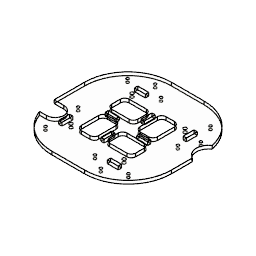
BasePlate_v8 (Autodesk Fusion 360 design; units mm, degrees)
Autodesk Fusion 360 part; units mm, degrees
sketch "Sketch1" plane through (0, 0, 0) normal (0, 0, 1) x (1, 0, 0)
  line L0 (-33.4, -17.4) -> (-33.4, 33.4) construction
  line L1 (-33.4, 33.4) -> (-27.4, 33.4) construction
  line L2 (-33.4, -17.4) -> (-36.4, -17.4)
  line L3 (-36.4, -17.4) -> (-36.4, -27.4)
  line L4 (-36.4, -27.4) -> (-33.4, -27.4)
  line L5 (-33.4, -27.4) -> (-33.4, -17.4)
  line L6 (-27.4, 33.4) -> (-17.4, 33.4)
  line L7 (-17.4, 33.4) -> (-17.4, 36.4)
  line L8 (-17.4, 36.4) -> (-27.4, 36.4)
  line L9 (-27.4, 36.4) -> (-27.4, 33.4)
  line L10 (-17.4, 33.4) -> (33.4, 33.4) construction
  line L11 (33.4, 33.4) -> (33.4, 27.4) construction
  line L12 (33.4, 27.4) -> (36.4, 27.4)
  line L13 (36.4, 27.4) -> (36.4, 17.4)
  line L14 (36.4, 17.4) -> (33.4, 17.4)
  line L15 (33.4, 17.4) -> (33.4, 27.4)
  line L16 (33.4, 17.4) -> (33.4, -33.4) construction
  line L17 (33.4, -33.4) -> (27.4, -33.4) construction
  line L18 (27.4, -33.4) -> (17.4, -33.4)
  line L19 (17.4, -33.4) -> (17.4, -36.4)
  line L20 (17.4, -36.4) -> (27.4, -36.4)
  line L21 (27.4, -36.4) -> (27.4, -33.4)
  line L22 (17.4, -33.4) -> (-33.4, -33.4) construction
  line L23 (-33.4, -33.4) -> (-33.4, -27.4) construction
  line L24 (33.4, 33.4) -> (-33.4, -33.4) construction
  line L25 (33.4, -33.4) -> (-33.4, 33.4) construction
  line L26 (55, -55) -> (-55, -55)
  line L27 (-55, -55) -> (-55, 55)
  line L28 (-55, 55) -> (55, 55)
  line L29 (55, 55) -> (55, -55)
  line L30 (55, -55) -> (-55, 55) construction
  line L31 (-55, -55) -> (55, 55) construction
  line L32 (-34.9, -17.4) -> (-34.9, -7.75) construction
  line L33 (-34.9, -7.75) -> (-38.15, -7.75) construction
  circle A0 centre (-38.15, -7.75) radius 1.25
  line L34 (-34.9, -27.4) -> (-34.9, -38.15) construction
  line L35 (-34.9, -38.15) -> (-37.75, -38.15) construction
  circle A1 centre (-37.75, -38.15) radius 1.25
  circle A2 centre (38.15, -37.75) radius 1.25
  circle A3 centre (7.75, -38.15) radius 1.25
  circle A4 centre (37.75, 38.15) radius 1.25
  circle A5 centre (38.15, 7.75) radius 1.25
  circle A6 centre (-38.15, 37.75) radius 1.25
  circle A7 centre (-7.75, 38.15) radius 1.25
  line L36 (0, 0) -> (0, 11.5) construction
  line L37 (0, 11.5) -> (3.5, 11.5) construction
  line L38 (3.5, 11.5) -> (0.5, 11.5)
  line L39 (0.5, 11.5) -> (0.5, 21.5)
  line L40 (0.5, 21.5) -> (3.5, 21.5)
  line L41 (3.5, 21.5) -> (3.5, 11.5)
  line L42 (-21.5, 3.5) -> (-11.5, 3.5)
  line L43 (-21.5, 0.5) -> (-21.5, 3.5)
  line L44 (-11.5, 0.5) -> (-21.5, 0.5)
  line L45 (-11.5, 3.5) -> (-11.5, 0.5)
  line L46 (-3.5, -21.5) -> (-3.5, -11.5)
  line L47 (-0.5, -21.5) -> (-3.5, -21.5)
  line L48 (-0.5, -11.5) -> (-0.5, -21.5)
  line L49 (-3.5, -11.5) -> (-0.5, -11.5)
  line L50 (21.5, -3.5) -> (11.5, -3.5)
  line L51 (21.5, -0.5) -> (21.5, -3.5)
  line L52 (11.5, -0.5) -> (21.5, -0.5)
  line L53 (11.5, -3.5) -> (11.5, -0.5)
  circle A8 centre (-24.4, 28.1) radius 1.5
  circle A9 centre (-28.1, -24.4) radius 1.5
  circle A10 centre (24.4, -28.1) radius 1.5
  circle A11 centre (28.1, 24.4) radius 1.5
  dimension "d1" = 50.8
  dimension "d2" = 6
  dimension "d3" = 3
  dimension "d4" = 10
  dimension "d5" = 10
  dimension "d6" = 3
  dimension "d7" = 50.8
  dimension "d8" = 6
  dimension "d9" = 3
  dimension "d10" = 10
  dimension "d11" = 50.8
  dimension "d12" = 6
  dimension "d13" = 10
  dimension "d14" = 3
  dimension "d15" = 50.8
  dimension "d16" = 110
  dimension "d17" = 110
  dimension "d22" = 9.65
  dimension "d23" = 3.25
  dimension "d24" = 2.5
  dimension "d25" = 10.75
  dimension "d26" = 2.85
  dimension "d27" = 2.5
  dimension "d29" = 360
  dimension "d34" = 11.5
  dimension "d36" = 3
  dimension "d37" = 10
  dimension "d39" = 360
  dimension "d40" = 0.5
  dimension "d41" = 3
  dimension "d43" = 360
  constraint vertical L0
  constraint perpendicular L0 L1
  constraint horizontal L2
  constraint vertical L3
  constraint horizontal L4
  constraint vertical L5
  constraint horizontal L6
  constraint vertical L7
  constraint horizontal L8
  constraint vertical L9
  constraint perpendicular L7 L10
  constraint perpendicular L10 L11
  constraint horizontal L12
  constraint vertical L13
  constraint horizontal L14
  constraint vertical L15
  constraint perpendicular L14 L16
  constraint perpendicular L16 L17
  constraint horizontal L18
  constraint vertical L19
  constraint horizontal L20
  constraint vertical L21
  constraint perpendicular L19 L22
  constraint coincident L36.start L24
  constraint coincident L36.start L25
  constraint horizontal L26
  constraint perpendicular L26 L27
  constraint parallel L26 L28
  constraint parallel L27 L29
  constraint coincident L30 L36.start
  constraint coincident L31 L36.start
  constraint coincident L36.start origin
  constraint midpoint L2 L32.start
  constraint perpendicular L2 L32
  constraint perpendicular L32 L33
  constraint coincident L33.end A0.centre
  constraint midpoint L4 L34.start
  constraint perpendicular L4 L34
  constraint perpendicular L34 L35
  constraint coincident L35.end A1.centre
  constraint vertical L36
  constraint horizontal L37
  constraint horizontal L38
  constraint vertical L39
  constraint horizontal L40
  constraint vertical L41
  measures "d1" distance of L0.start L0.end
  measures "d2" distance of L0.end L1.end
  measures "d3" distance of L0.start L2.end
  measures "d4" distance of L0.start L4.end
  measures "d5" distance of L1.end L6.end
  measures "d6" distance of L1.end L8.end
  measures "d7" distance of L6.end L10.end
  measures "d8" distance of L10.end L11.end
  measures "d9" distance of L11.end L12.end
  measures "d10" distance of L11.end L14.end
  measures "d11" distance of L14.end L16.end
  measures "d12" distance of L16.end L17.end
  measures "d13" distance of L17.end L18.end
  measures "d14" distance of L17.end L20.end
  measures "d15" distance of L18.end L22.end
  measures "d16" distance of L27.end L28.end
  measures "d17" distance of L26.end L27.end
  measures "d22" distance of L32.start L32.end
  measures "d23" distance of L32.end L33.end
  measures "d24" diameter of A0
  measures "d25" distance of L34.start L34.end
  measures "d26" distance of L34.end L35.end
  measures "d27" diameter of A1
  measures "d34" distance of L36.start L36.end
  measures "d36" distance of L37.end L38.end
  measures "d37" distance of L37.end L40.end
  measures "d40" distance of L36 L39
  measures "d41" diameter of A8
extrude "Extrude1" add sketch "Sketch1" along normal blind 3 contours L26 L27 L28 L29 | A0 | A1 | A2 | A3 | A4 | A5 | A6 | A7 | L38 L39 L40 L41 | L42 L43 L44 L45 | L46 L47 L48 L49 | L50 L51 L52 L53 | A8 | A9 | A10 | A11
extrude "Extrude2" cut sketch "Sketch1" along normal blind 3 contours A0 | A1 | A2 | A3 | A4 | A5 | A6 | A7 | L38 L39 L40 L41 | L42 L43 L44 L45 | L46 L47 L48 L49 | L50 L51 L52 L53
fillet "Fillet1" radius 40 4 edges at (55, -55, 1.5) (-55, -55, 1.5) (55, 55, 1.5) (-55, 55, 1.5)
extrude "Extrude3" cut sketch "Sketch1" along normal blind 14 contours A8 | A9 | A10 | A11
sketch "Sketch2" plane through (0, 0, 3) normal (0, 0, 1) x (-1, 0, 0)
  line L0 (11.5, -3.5) -> (11.5, -0.5)
  line L1 (11.5, -0.5) -> (21.5, -0.5)
  line L2 (21.5, -0.5) -> (21.5, -3.5)
  line L3 (21.5, -3.5) -> (11.5, -3.5)
  circle A0 centre (-7.75, 38.15) radius 1.25
  circle A1 centre (7.75, -38.15) radius 1.25
  circle A2 centre (-37.75, -38.15) radius 1.25
  circle A3 centre (37.75, 38.15) radius 1.25
  line L4 (3.5, 11.5) -> (0.5, 11.5)
  line L5 (0.5, 11.5) -> (0.5, 21.5)
  line L6 (0.5, 21.5) -> (3.5, 21.5)
  line L7 (3.5, 21.5) -> (3.5, 11.5)
  line L8 (-3.5, -21.5) -> (-3.5, -11.5)
  line L9 (-3.5, -11.5) -> (-0.5, -11.5)
  line L10 (-0.5, -11.5) -> (-0.5, -21.5)
  line L11 (-0.5, -21.5) -> (-3.5, -21.5)
  circle A4 centre (-38.15, 37.75) radius 1.25
  circle A5 centre (38.15, -37.75) radius 1.25
  circle A6 centre (-38.15, -7.75) radius 1.25
  circle A7 centre (38.15, 7.75) radius 1.25
  line L12 (-11.5, 3.5) -> (-11.5, 0.5)
  line L13 (-11.5, 0.5) -> (-21.5, 0.5)
  line L14 (-21.5, 0.5) -> (-21.5, 3.5)
  line L15 (-21.5, 3.5) -> (-11.5, 3.5)
  line L16 (-36.4, -17.4) -> (-33.4, -17.4)
  line L17 (-33.4, -17.4) -> (-33.4, -27.4)
  line L18 (-33.4, -27.4) -> (-36.4, -27.4)
  line L19 (-36.4, -27.4) -> (-36.4, -17.4)
  line L20 (27.4, -33.4) -> (27.4, -36.4)
  line L21 (27.4, -36.4) -> (17.4, -36.4)
  line L22 (17.4, -36.4) -> (17.4, -33.4)
  line L23 (17.4, -33.4) -> (27.4, -33.4)
  line L24 (33.4, 17.4) -> (33.4, 27.4)
  line L25 (33.4, 27.4) -> (36.4, 27.4)
  line L26 (36.4, 27.4) -> (36.4, 17.4)
  line L27 (36.4, 17.4) -> (33.4, 17.4)
  line L28 (-27.4, 33.4) -> (-27.4, 36.4)
  line L29 (-27.4, 36.4) -> (-17.4, 36.4)
  line L30 (-17.4, 36.4) -> (-17.4, 33.4)
  line L31 (-17.4, 33.4) -> (-27.4, 33.4)
  arc A8 (15, -55) -> (55, -15) centre (15, -15) ccw
  line L32 (55, -15) -> (55, 15)
  arc A9 (55, 15) -> (15, 55) centre (15, 15) ccw
  line L33 (15, 55) -> (-15, 55)
  arc A10 (-15, 55) -> (-55, 15) centre (-15, 15) ccw
  line L34 (-55, 15) -> (-55, -15)
  arc A11 (-55, -15) -> (-15, -55) centre (-15, -15) ccw
  line L35 (-15, -55) -> (15, -55)
  circle A12 centre (-24.4, 28.1) radius 1.5
  circle A13 centre (-28.1, -24.4) radius 1.5
  circle A14 centre (28.1, 24.4) radius 1.5
  circle A15 centre (24.4, -28.1) radius 1.5
  line L36 (-1, 22) -> (-25, 22)
  line L37 (-25, 22) -> (-25, 6)
  line L38 (-25, 6) -> (-1, 6)
  line L39 (-1, 6) -> (-1, 22)
  line L40 (-22, -1) -> (-22, -25)
  line L41 (-22, -25) -> (-6, -25)
  line L42 (-6, -1) -> (-22, -1)
  line L43 (-6, -25) -> (-6, -1)
  line L44 (1, -22) -> (25, -22)
  line L45 (25, -22) -> (25, -6)
  line L46 (1, -6) -> (1, -22)
  line L47 (25, -6) -> (1, -6)
  line L48 (22, 1) -> (22, 25)
  line L49 (22, 25) -> (6, 25)
  line L50 (6, 1) -> (22, 1)
  line L51 (6, 25) -> (6, 1)
  dimension "d47" = 360
  constraint horizontal L36
  constraint vertical L37
  constraint horizontal L38
  constraint vertical L39
extrude "Extrude4" cut sketch "Sketch2" against normal blind 5 contours L36 L37 L38 L39 | L40 L41 L42 L43 | L44 L45 L46 L47 | L48 L49 L50 L51
fillet "Fillet2" radius 4 16 edges at (25, -22, 1.5) (25, -6, 1.5) (1, -22, 1.5) (1, -6, 1.5) (-6, -25, 1.5) (-22, -25, 1.5) (-22, -1, 1.5) (-6, -1, 1.5) (-25, 6, 1.5) (-25, 22, 1.5) (-1, 22, 1.5) (-1, 6, 1.5) (22, 1, 1.5) (6, 1, 1.5) (6, 25, 1.5) (22, 25, 1.5)
sketch "Sketch3" plane through (0, 0, 3) normal (0, 0, 1) x (-1, 0, 0)
  circle A0 centre (24.4, -28.1) radius 1.5
  circle A1 centre (28.1, 24.4) radius 1.5
  circle A2 centre (-28.1, -24.4) radius 1.5
  circle A3 centre (-24.4, 28.1) radius 1.5
  arc A4 (15, -55) -> (55, -15) centre (15, -15) ccw
  line L0 (55, -15) -> (55, 15)
  arc A5 (55, 15) -> (15, 55) centre (15, 15) ccw
  line L1 (15, 55) -> (-15, 55)
  arc A6 (-15, 55) -> (-55, 15) centre (-15, 15) ccw
  line L2 (-55, 15) -> (-55, -15)
  arc A7 (-55, -15) -> (-15, -55) centre (-15, -15) ccw
  line L3 (-15, -55) -> (15, -55)
  line L4 (-27.4, 33.4) -> (-27.4, 36.4)
  line L5 (-27.4, 36.4) -> (-17.4, 36.4)
  line L6 (-17.4, 36.4) -> (-17.4, 33.4)
  line L7 (-17.4, 33.4) -> (-27.4, 33.4)
  line L8 (33.4, 17.4) -> (33.4, 27.4)
  line L9 (33.4, 27.4) -> (36.4, 27.4)
  line L10 (36.4, 27.4) -> (36.4, 17.4)
  line L11 (36.4, 17.4) -> (33.4, 17.4)
  line L12 (27.4, -33.4) -> (27.4, -36.4)
  line L13 (27.4, -36.4) -> (17.4, -36.4)
  line L14 (17.4, -36.4) -> (17.4, -33.4)
  line L15 (17.4, -33.4) -> (27.4, -33.4)
  line L16 (-36.4, -17.4) -> (-33.4, -17.4)
  line L17 (-33.4, -17.4) -> (-33.4, -27.4)
  line L18 (-33.4, -27.4) -> (-36.4, -27.4)
  line L19 (-36.4, -27.4) -> (-36.4, -17.4)
  line L20 (-11.5, 3.5) -> (-11.5, 0.5)
  line L21 (-11.5, 0.5) -> (-21.5, 0.5)
  line L22 (-21.5, 0.5) -> (-21.5, 3.5)
  line L23 (-21.5, 3.5) -> (-11.5, 3.5)
  circle A8 centre (38.15, 7.75) radius 1.25
  circle A9 centre (-38.15, -7.75) radius 1.25
  circle A10 centre (38.15, -37.75) radius 1.25
  circle A11 centre (-38.15, 37.75) radius 1.25
  line L24 (-3.5, -21.5) -> (-3.5, -11.5)
  line L25 (-3.5, -11.5) -> (-0.5, -11.5)
  line L26 (-0.5, -11.5) -> (-0.5, -21.5)
  line L27 (-0.5, -21.5) -> (-3.5, -21.5)
  line L28 (3.5, 11.5) -> (0.5, 11.5)
  line L29 (0.5, 11.5) -> (0.5, 21.5)
  line L30 (0.5, 21.5) -> (3.5, 21.5)
  line L31 (3.5, 21.5) -> (3.5, 11.5)
  circle A12 centre (37.75, 38.15) radius 1.25
  circle A13 centre (-37.75, -38.15) radius 1.25
  circle A14 centre (7.75, -38.15) radius 1.25
  circle A15 centre (-7.75, 38.15) radius 1.25
  line L32 (11.5, -3.5) -> (11.5, -0.5)
  line L33 (11.5, -0.5) -> (21.5, -0.5)
  line L34 (21.5, -0.5) -> (21.5, -3.5)
  line L35 (21.5, -3.5) -> (11.5, -3.5)
  line L36 (-21, 22) -> (-5, 22)
  arc A16 (-1, 18) -> (-5, 22) centre (-5, 18) ccw
  line L37 (-1, 18) -> (-1, 10)
  arc A17 (-5, 6) -> (-1, 10) centre (-5, 10) ccw
  line L38 (-5, 6) -> (-21, 6)
  arc A18 (-25, 10) -> (-21, 6) centre (-21, 10) ccw
  line L39 (-25, 10) -> (-25, 18)
  arc A19 (-21, 22) -> (-25, 18) centre (-21, 18) ccw
  line L40 (-18, -1) -> (-10, -1)
  arc A20 (-6, -5) -> (-10, -1) centre (-10, -5) ccw
  line L41 (-6, -5) -> (-6, -21)
  arc A21 (-10, -25) -> (-6, -21) centre (-10, -21) ccw
  line L42 (-10, -25) -> (-18, -25)
  arc A22 (-22, -21) -> (-18, -25) centre (-18, -21) ccw
  line L43 (-22, -21) -> (-22, -5)
  arc A23 (-18, -1) -> (-22, -5) centre (-18, -5) ccw
  line L44 (18, 1) -> (10, 1)
  arc A24 (6, 5) -> (10, 1) centre (10, 5) ccw
  line L45 (6, 5) -> (6, 21)
  arc A25 (10, 25) -> (6, 21) centre (10, 21) ccw
  line L46 (10, 25) -> (18, 25)
  arc A26 (22, 21) -> (18, 25) centre (18, 21) ccw
  line L47 (22, 21) -> (22, 5)
  arc A27 (18, 1) -> (22, 5) centre (18, 5) ccw
  line L48 (1, -18) -> (1, -10)
  arc A28 (5, -6) -> (1, -10) centre (5, -10) ccw
  line L49 (5, -6) -> (21, -6)
  arc A29 (25, -10) -> (21, -6) centre (21, -10) ccw
  line L50 (25, -10) -> (25, -18)
  arc A30 (21, -22) -> (25, -18) centre (21, -18) ccw
  line L51 (21, -22) -> (5, -22)
  arc A31 (1, -18) -> (5, -22) centre (5, -18) ccw
  circle A32 centre (21.0277, -45.9989) radius 8
  line L52 (21.0277, -45.9989) -> (13.0277, -45.9989) construction
  line L53 (13.0277, -45.9989) -> (13.0277, -54.9513)
  line L54 (21.0277, -45.9989) -> (29.0277, -45.9989) construction
  line L55 (29.0277, -45.9989) -> (29.0277, -52.4596)
  line L56 (13.0277, -54.9513) -> (13.0277, -55.3585)
  line L57 (45.9989, 29.0277) -> (52.4596, 29.0277)
  circle A33 centre (45.9989, 21.0277) radius 8
  line L58 (45.9989, 13.0277) -> (54.9513, 13.0277)
  line L59 (-29.0277, 45.9989) -> (-29.0277, 52.4596)
  circle A34 centre (-21.0277, 45.9989) radius 8
  line L60 (-13.0277, 45.9989) -> (-13.0277, 54.9513)
  line L61 (-45.9989, -29.0277) -> (-52.4596, -29.0277)
  circle A35 centre (-45.9989, -21.0277) radius 8
  line L62 (-45.9989, -13.0277) -> (-54.9513, -13.0277)
  line L63 (54.9513, 13.0277) -> (55, 13.0277)
  dimension "d52" = 16
  dimension "d58" = 360
  constraint coincident A32.centre L52.start
  constraint coincident A32 L52.end
  constraint horizontal L52
  constraint coincident A4 L53.end
  constraint tangent A32 L53
  constraint coincident A32 L54.end
  constraint perpendicular L53 L54
  constraint coincident A4 L55.end
  constraint tangent A32 L55
  constraint perpendicular L3 L56
  constraint coincident L0 L63.end
  constraint perpendicular L0 L63
  measures "d52" diameter of A32
extrude "Extrude5" cut sketch "Sketch3" against normal blind 8 contours L0 A5 L57 A33 L58 L63 | A33
sketch "Sketch4" plane through (0, 0, 3) normal (0, 0, 1) x (-1, 0, 0)
  arc A0 (15, -55) -> (55, -15) centre (15, -15) ccw
  line L0 (55, -15) -> (55, 13.0277)
  arc A1 (52.4596, 29.0277) -> (15, 55) centre (15, 15) ccw
  line L1 (15, 55) -> (-15, 55)
  arc A2 (-15, 55) -> (-55, 15) centre (-15, 15) ccw
  line L2 (-55, 15) -> (-55, -15)
  arc A3 (-55, -15) -> (-15, -55) centre (-15, -15) ccw
  line L3 (-15, -55) -> (15, -55)
  line L4 (1, -18) -> (1, -10)
  arc A4 (5, -6) -> (1, -10) centre (5, -10) ccw
  line L5 (5, -6) -> (21, -6)
  arc A5 (25, -10) -> (21, -6) centre (21, -10) ccw
  line L6 (25, -10) -> (25, -18)
  arc A6 (21, -22) -> (25, -18) centre (21, -18) ccw
  line L7 (21, -22) -> (5, -22)
  arc A7 (1, -18) -> (5, -22) centre (5, -18) ccw
  line L8 (18, 1) -> (10, 1)
  arc A8 (6, 5) -> (10, 1) centre (10, 5) ccw
  line L9 (6, 5) -> (6, 21)
  arc A9 (10, 25) -> (6, 21) centre (10, 21) ccw
  line L10 (10, 25) -> (18, 25)
  arc A10 (22, 21) -> (18, 25) centre (18, 21) ccw
  line L11 (22, 21) -> (22, 5)
  arc A11 (18, 1) -> (22, 5) centre (18, 5) ccw
  line L12 (-18, -1) -> (-10, -1)
  arc A12 (-6, -5) -> (-10, -1) centre (-10, -5) ccw
  line L13 (-6, -5) -> (-6, -21)
  arc A13 (-10, -25) -> (-6, -21) centre (-10, -21) ccw
  line L14 (-10, -25) -> (-18, -25)
  arc A14 (-22, -21) -> (-18, -25) centre (-18, -21) ccw
  line L15 (-22, -21) -> (-22, -5)
  arc A15 (-18, -1) -> (-22, -5) centre (-18, -5) ccw
  line L16 (-21, 22) -> (-5, 22)
  arc A16 (-1, 18) -> (-5, 22) centre (-5, 18) ccw
  line L17 (-1, 18) -> (-1, 10)
  arc A17 (-5, 6) -> (-1, 10) centre (-5, 10) ccw
  line L18 (-5, 6) -> (-21, 6)
  arc A18 (-25, 10) -> (-21, 6) centre (-21, 10) ccw
  line L19 (-25, 10) -> (-25, 18)
  arc A19 (-21, 22) -> (-25, 18) centre (-21, 18) ccw
  line L20 (11.5, -3.5) -> (11.5, -0.5)
  line L21 (11.5, -0.5) -> (21.5, -0.5)
  line L22 (21.5, -0.5) -> (21.5, -3.5)
  line L23 (21.5, -3.5) -> (11.5, -3.5)
  circle A20 centre (-7.75, 38.15) radius 1.25
  circle A21 centre (7.75, -38.15) radius 1.25
  circle A22 centre (-37.75, -38.15) radius 1.25
  circle A23 centre (37.75, 38.15) radius 1.25
  line L24 (3.5, 11.5) -> (0.5, 11.5)
  line L25 (0.5, 11.5) -> (0.5, 21.5)
  line L26 (0.5, 21.5) -> (3.5, 21.5)
  line L27 (3.5, 21.5) -> (3.5, 11.5)
  line L28 (-3.5, -21.5) -> (-3.5, -11.5)
  line L29 (-3.5, -11.5) -> (-0.5, -11.5)
  line L30 (-0.5, -11.5) -> (-0.5, -21.5)
  line L31 (-0.5, -21.5) -> (-3.5, -21.5)
  circle A24 centre (-38.15, 37.75) radius 1.25
  circle A25 centre (38.15, -37.75) radius 1.25
  circle A26 centre (-38.15, -7.75) radius 1.25
  circle A27 centre (38.15, 7.75) radius 1.25
  line L32 (-11.5, 3.5) -> (-11.5, 0.5)
  line L33 (-11.5, 0.5) -> (-21.5, 0.5)
  line L34 (-21.5, 0.5) -> (-21.5, 3.5)
  line L35 (-21.5, 3.5) -> (-11.5, 3.5)
  line L36 (-36.4, -17.4) -> (-33.4, -17.4)
  line L37 (-33.4, -17.4) -> (-33.4, -27.4)
  line L38 (-33.4, -27.4) -> (-36.4, -27.4)
  line L39 (-36.4, -27.4) -> (-36.4, -17.4)
  line L40 (27.4, -33.4) -> (27.4, -36.4)
  line L41 (27.4, -36.4) -> (17.4, -36.4)
  line L42 (17.4, -36.4) -> (17.4, -33.4)
  line L43 (17.4, -33.4) -> (27.4, -33.4)
  line L44 (33.4, 17.4) -> (33.4, 27.4)
  line L45 (33.4, 27.4) -> (36.4, 27.4)
  line L46 (36.4, 27.4) -> (36.4, 17.4)
  line L47 (36.4, 17.4) -> (33.4, 17.4)
  line L48 (-27.4, 33.4) -> (-27.4, 36.4)
  line L49 (-27.4, 36.4) -> (-17.4, 36.4)
  line L50 (-17.4, 36.4) -> (-17.4, 33.4)
  line L51 (-17.4, 33.4) -> (-27.4, 33.4)
  circle A28 centre (-24.4, 28.1) radius 1.5
  circle A29 centre (-28.1, -24.4) radius 1.5
  circle A30 centre (28.1, 24.4) radius 1.5
  circle A31 centre (24.4, -28.1) radius 1.5
  circle A32 centre (-21.0277, 45.9989) radius 1.25
  circle A33 centre (45.9989, 21.0277) radius 1.25
  circle A34 centre (-45.9989, -21.0277) radius 1.25
  circle A35 centre (21.0277, -45.9989) radius 1.25
  line L52 (45.9989, 29.0277) -> (52.4596, 29.0277)
  line L53 (55, 13.0277) -> (45.9989, 13.0277)
  arc A36 (45.9989, 29.0277) -> (45.9989, 13.0277) centre (45.9989, 21.0277) ccw
extrude "Extrude6" cut sketch "Sketch4" against normal blind 15 contours A32 | A33 | A34
sketch "Laser" plane through (0, 0, 3) normal (0, 0, 1) x (-1, 0, 0)
  circle A0 centre (24.4, -28.1) radius 1.5
  circle A1 centre (28.1, 24.4) radius 1.5
  circle A2 centre (-28.1, -24.4) radius 1.5
  circle A3 centre (-24.4, 28.1) radius 1.5
  line L0 (-27.4, 33.4) -> (-27.4, 36.4)
  line L1 (-27.4, 36.4) -> (-17.4, 36.4)
  line L2 (-17.4, 36.4) -> (-17.4, 33.4)
  line L3 (-17.4, 33.4) -> (-27.4, 33.4)
  line L4 (33.4, 17.4) -> (33.4, 27.4)
  line L5 (33.4, 27.4) -> (36.4, 27.4)
  line L6 (36.4, 27.4) -> (36.4, 17.4)
  line L7 (36.4, 17.4) -> (33.4, 17.4)
  line L8 (27.4, -33.4) -> (27.4, -36.4)
  line L9 (27.4, -36.4) -> (17.4, -36.4)
  line L10 (17.4, -36.4) -> (17.4, -33.4)
  line L11 (17.4, -33.4) -> (27.4, -33.4)
  line L12 (-36.4, -17.4) -> (-33.4, -17.4)
  line L13 (-33.4, -17.4) -> (-33.4, -27.4)
  line L14 (-33.4, -27.4) -> (-36.4, -27.4)
  line L15 (-36.4, -27.4) -> (-36.4, -17.4)
  line L16 (-11.5, 3.5) -> (-11.5, 0.5)
  line L17 (-11.5, 0.5) -> (-21.5, 0.5)
  line L18 (-21.5, 0.5) -> (-21.5, 3.5)
  line L19 (-21.5, 3.5) -> (-11.5, 3.5)
  circle A4 centre (38.15, 7.75) radius 1.25
  circle A5 centre (-38.15, -7.75) radius 1.25
  circle A6 centre (38.15, -37.75) radius 1.25
  circle A7 centre (-38.15, 37.75) radius 1.25
  line L20 (-3.5, -21.5) -> (-3.5, -11.5)
  line L21 (-3.5, -11.5) -> (-0.5, -11.5)
  line L22 (-0.5, -11.5) -> (-0.5, -21.5)
  line L23 (-0.5, -21.5) -> (-3.5, -21.5)
  line L24 (3.5, 11.5) -> (0.5, 11.5)
  line L25 (0.5, 11.5) -> (0.5, 21.5)
  line L26 (0.5, 21.5) -> (3.5, 21.5)
  line L27 (3.5, 21.5) -> (3.5, 11.5)
  circle A8 centre (37.75, 38.15) radius 1.25
  circle A9 centre (-37.75, -38.15) radius 1.25
  circle A10 centre (7.75, -38.15) radius 1.25
  circle A11 centre (-7.75, 38.15) radius 1.25
  line L28 (11.5, -3.5) -> (11.5, -0.5)
  line L29 (11.5, -0.5) -> (21.5, -0.5)
  line L30 (21.5, -0.5) -> (21.5, -3.5)
  line L31 (21.5, -3.5) -> (11.5, -3.5)
  line L32 (-21, 22) -> (-5, 22)
  arc A12 (-1, 18) -> (-5, 22) centre (-5, 18) ccw
  line L33 (-1, 18) -> (-1, 10)
  arc A13 (-5, 6) -> (-1, 10) centre (-5, 10) ccw
  line L34 (-5, 6) -> (-21, 6)
  arc A14 (-25, 10) -> (-21, 6) centre (-21, 10) ccw
  line L35 (-25, 10) -> (-25, 18)
  arc A15 (-21, 22) -> (-25, 18) centre (-21, 18) ccw
  line L36 (-18, -1) -> (-10, -1)
  arc A16 (-6, -5) -> (-10, -1) centre (-10, -5) ccw
  line L37 (-6, -5) -> (-6, -21)
  arc A17 (-10, -25) -> (-6, -21) centre (-10, -21) ccw
  line L38 (-10, -25) -> (-18, -25)
  arc A18 (-22, -21) -> (-18, -25) centre (-18, -21) ccw
  line L39 (-22, -21) -> (-22, -5)
  arc A19 (-18, -1) -> (-22, -5) centre (-18, -5) ccw
  line L40 (18, 1) -> (10, 1)
  arc A20 (6, 5) -> (10, 1) centre (10, 5) ccw
  line L41 (6, 5) -> (6, 21)
  arc A21 (10, 25) -> (6, 21) centre (10, 21) ccw
  line L42 (10, 25) -> (18, 25)
  arc A22 (22, 21) -> (18, 25) centre (18, 21) ccw
  line L43 (22, 21) -> (22, 5)
  arc A23 (18, 1) -> (22, 5) centre (18, 5) ccw
  line L44 (1, -18) -> (1, -10)
  arc A24 (5, -6) -> (1, -10) centre (5, -10) ccw
  line L45 (5, -6) -> (21, -6)
  arc A25 (25, -10) -> (21, -6) centre (21, -10) ccw
  line L46 (25, -10) -> (25, -18)
  arc A26 (21, -22) -> (25, -18) centre (21, -18) ccw
  line L47 (21, -22) -> (5, -22)
  arc A27 (1, -18) -> (5, -22) centre (5, -18) ccw
  arc A28 (15, -55) -> (55, -15) centre (15, -15) ccw
  line L48 (55, -15) -> (55, 13.0277)
  arc A29 (52.4596, 29.0277) -> (15, 55) centre (15, 15) ccw
  line L49 (15, 55) -> (-15, 55)
  arc A30 (-15, 55) -> (-55, 15) centre (-15, 15) ccw
  line L50 (-55, 15) -> (-55, -15)
  arc A31 (-55, -15) -> (-15, -55) centre (-15, -15) ccw
  line L51 (-15, -55) -> (15, -55)
  circle A32 centre (-45.9989, -21.0277) radius 1.25
  circle A33 centre (-21.0277, 45.9989) radius 1.25
  line L52 (45.9989, 29.0277) -> (52.4596, 29.0277)
  line L53 (55, 13.0277) -> (45.9989, 13.0277)
  arc A34 (45.9989, 29.0277) -> (45.9989, 13.0277) centre (45.9989, 21.0277) ccw
extrude "Extrude7" cut sketch "Sketch4" against normal blind 9 contours A35
sketch "Sketch6" plane through (0, 0, 0) normal (0, 0, -1) x (1, 0, 0)
  circle A0 centre (21.0277, 45.9989) radius 1.25
  circle A1 centre (45.9989, -21.0277) radius 1.25
  line L0 (-52.4596, 29.0277) -> (-45.9989, 29.0277)
  arc A2 (-45.9989, 13.0277) -> (-45.9989, 29.0277) centre (-45.9989, 21.0277) ccw
  line L1 (-45.9989, 13.0277) -> (-55, 13.0277)
  line L2 (-55, 13.0277) -> (-55, -15)
  arc A3 (-55, -15) -> (-15, -55) centre (-15, -15) ccw
  line L3 (-15, -55) -> (15, -55)
  arc A4 (15, -55) -> (55, -15) centre (15, -15) ccw
  line L4 (55, -15) -> (55, 15)
  arc A5 (55, 15) -> (15, 55) centre (15, 15) ccw
  line L5 (15, 55) -> (-15, 55)
  arc A6 (-15, 55) -> (-52.4596, 29.0277) centre (-15, 15) ccw
  line L6 (-1, -10) -> (-1, -18)
  arc A7 (-5, -22) -> (-1, -18) centre (-5, -18) ccw
  line L7 (-5, -22) -> (-21, -22)
  arc A8 (-25, -18) -> (-21, -22) centre (-21, -18) ccw
  line L8 (-25, -18) -> (-25, -10)
  arc A9 (-21, -6) -> (-25, -10) centre (-21, -10) ccw
  line L9 (-21, -6) -> (-5, -6)
  arc A10 (-1, -10) -> (-5, -6) centre (-5, -10) ccw
  line L10 (-10, 1) -> (-18, 1)
  arc A11 (-22, 5) -> (-18, 1) centre (-18, 5) ccw
  line L11 (-22, 5) -> (-22, 21)
  arc A12 (-18, 25) -> (-22, 21) centre (-18, 21) ccw
  line L12 (-18, 25) -> (-10, 25)
  arc A13 (-6, 21) -> (-10, 25) centre (-10, 21) ccw
  line L13 (-6, 21) -> (-6, 5)
  arc A14 (-10, 1) -> (-6, 5) centre (-10, 5) ccw
  line L14 (10, -1) -> (18, -1)
  arc A15 (22, -5) -> (18, -1) centre (18, -5) ccw
  line L15 (22, -5) -> (22, -21)
  arc A16 (18, -25) -> (22, -21) centre (18, -21) ccw
  line L16 (18, -25) -> (10, -25)
  arc A17 (6, -21) -> (10, -25) centre (10, -21) ccw
  line L17 (6, -21) -> (6, -5)
  arc A18 (10, -1) -> (6, -5) centre (10, -5) ccw
  line L18 (5, 22) -> (21, 22)
  arc A19 (25, 18) -> (21, 22) centre (21, 18) ccw
  line L19 (25, 18) -> (25, 10)
  arc A20 (21, 6) -> (25, 10) centre (21, 10) ccw
  line L20 (21, 6) -> (5, 6)
  arc A21 (1, 10) -> (5, 6) centre (5, 10) ccw
  line L21 (1, 10) -> (1, 18)
  arc A22 (5, 22) -> (1, 18) centre (5, 18) ccw
  line L22 (-11.5, -0.5) -> (-11.5, -3.5)
  line L23 (-11.5, -3.5) -> (-21.5, -3.5)
  line L24 (-21.5, -3.5) -> (-21.5, -0.5)
  line L25 (-21.5, -0.5) -> (-11.5, -0.5)
  circle A23 centre (7.75, 38.15) radius 1.25
  circle A24 centre (-7.75, -38.15) radius 1.25
  circle A25 centre (37.75, -38.15) radius 1.25
  circle A26 centre (-37.75, 38.15) radius 1.25
  line L26 (-0.5, 11.5) -> (-3.5, 11.5)
  line L27 (-3.5, 11.5) -> (-3.5, 21.5)
  line L28 (-3.5, 21.5) -> (-0.5, 21.5)
  line L29 (-0.5, 21.5) -> (-0.5, 11.5)
  line L30 (3.5, -11.5) -> (3.5, -21.5)
  line L31 (3.5, -21.5) -> (0.5, -21.5)
  line L32 (0.5, -21.5) -> (0.5, -11.5)
  line L33 (0.5, -11.5) -> (3.5, -11.5)
  circle A27 centre (38.15, 37.75) radius 1.25
  circle A28 centre (-38.15, -37.75) radius 1.25
  circle A29 centre (38.15, -7.75) radius 1.25
  circle A30 centre (-38.15, 7.75) radius 1.25
  line L34 (11.5, 0.5) -> (11.5, 3.5)
  line L35 (11.5, 3.5) -> (21.5, 3.5)
  line L36 (21.5, 3.5) -> (21.5, 0.5)
  line L37 (21.5, 0.5) -> (11.5, 0.5)
  line L38 (33.4, -17.4) -> (36.4, -17.4)
  line L39 (36.4, -17.4) -> (36.4, -27.4)
  line L40 (36.4, -27.4) -> (33.4, -27.4)
  line L41 (33.4, -27.4) -> (33.4, -17.4)
  line L42 (-27.4, -36.4) -> (-27.4, -33.4)
  line L43 (-27.4, -33.4) -> (-17.4, -33.4)
  line L44 (-17.4, -33.4) -> (-17.4, -36.4)
  line L45 (-17.4, -36.4) -> (-27.4, -36.4)
  line L46 (-33.4, 27.4) -> (-33.4, 17.4)
  line L47 (-33.4, 17.4) -> (-36.4, 17.4)
  line L48 (-36.4, 17.4) -> (-36.4, 27.4)
  line L49 (-36.4, 27.4) -> (-33.4, 27.4)
  line L50 (27.4, 36.4) -> (27.4, 33.4)
  line L51 (27.4, 33.4) -> (17.4, 33.4)
  line L52 (17.4, 33.4) -> (17.4, 36.4)
  line L53 (17.4, 36.4) -> (27.4, 36.4)
  circle A31 centre (24.4, 28.1) radius 1.5
  circle A32 centre (28.1, -24.4) radius 1.5
  circle A33 centre (-28.1, 24.4) radius 1.5
  circle A34 centre (-24.4, -28.1) radius 1.5
  circle A35 centre (-21.0277, -45.9989) radius 1.25
  circle A36 centre (60, -14) radius 11
  dimension "d61" = 22
  measures "d61" diameter of A36
extrude "Extrude8" cut sketch "Sketch6" against normal blind 5 contours A4 L4 A36 | A4 L4 A36
